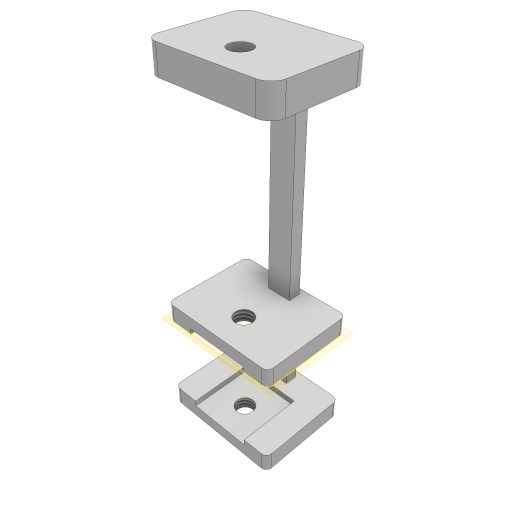
# Autodesk Inventor part: Crystal-Cut10x10-screwM4
Saved by Autodesk Inventor 2023 (Build 270158000, 158)
## iProperties
Created: 2021-08-04
Part Number: Crystal-Cut10x10-screwM4
Material: Generic
Document SubType Name: Modeling
Designer: Nikita
Density: 1 g/cm^3
Appearance: Default
Author: Nikita
Autodesk Inventor part; units mm, degrees
ref_plane "YZ Plane" through (0, 0, 0) normal (1, 0, 0) x (0, 1, 0)
ref_plane "XZ Plane" through (0, 0, 0) normal (0, 1, 0) x (-1, 0, 0)
ref_plane "XY Plane" through (0, 0, 0) normal (0, 0, 1) x (1, 0, 0)
sketch "Sketch1" plane through (0, 0, 0) normal (0, 0, 1) x (1, 0, 0)
  line L0 (0, 0) -> (19, 0)
  line L1 (19, 0) -> (19, 15)
  line L2 (19, 15) -> (0, 15)
  line L3 (0, 15) -> (0, 0)
  point P0 (9.5, 15)
  dimension "d0" = 19
  dimension "d1" = 15
  constraints: 8 end point, 2 parallel, 1 horizontal, 1 midpoint, 1 perpendicular
  measures "d0" distance of L2.end L1.end
  measures "d1" distance of L1.end L0.end
extrude "Extrusion1" add sketch "Sketch1" along normal blind 3
sketch "Sketch2" plane through (0, 0, 3) normal (0, 0, 1) x (1, 0, 0)
  line L0 (19, 15) -> (0, 15) projected
  circle A0 centre (9.5, 13) radius 1
  point P0 (0, 0)
  point P1 (9.5, 15)
  dimension "d4" = 2
  dimension "d5" = 2
  constraints: 1 centre point, 1 midpoint
  measures "d4" diameter of A0
  measures "d5" distance from line of A0.centre L0
extrude "Extrusion2" add sketch "Sketch2" along normal blind 1.5
sketch "Sketch6" plane through (9.5, 13, 4.5) normal (0, 0, 1) x (1, 0, 0)
  circle A0 centre (0, 0) radius 1 projected
  line L0 (2, -1) -> (-2, -1)
  line L1 (-2, -1) -> (-2, 1)
  line L2 (-2, 1) -> (2, 1)
  line L3 (2, 1) -> (2, -1)
  line L4 (2, -1) -> (-2, 1) construction
  line L5 (-2, -1) -> (2, 1) construction
  point P0 (-9.5, -13)
  dimension "d13" = 4
  constraints: 12 end point, 2 midpoint, 2 parallel, 1 coincident, 1 horizontal, 1 perpendicular
  measures "d13" distance of L1.end L2.end
extrude "Extrusion5" add sketch "Sketch6" along normal blind 47
sketch "Sketch7" plane through (9.5, 13, 51.5) normal (0, 0, 1) x (1, 0, 0)
  circle A0 centre (0, 0) radius 1 projected
  line L0 (-9.5, -13) -> (9.5, -13) projected
  line L1 (9.5, -13) -> (9.5, 2) projected
  line L2 (9.5, 2) -> (-9.5, 2) projected
  line L3 (-9.5, 2) -> (-9.5, -13) projected
  arc A1 (0, -1) -> (0, 1) centre (0, 0) ccw projected
  arc A2 (0, 1) -> (0, -1) centre (0, 0) ccw projected
extrude "Extrusion6" add sketch "Sketch7" along normal blind 4 contours A0 | L3 L2 L1 L0
fillet "Fillet2" radius 1 4 edges at (19, 0, 1.5) (19, 15, 1.5) (0, 0, 1.5) (0, 15, 1.5)
fillet "Fillet3" radius 2 4 edges at (19, 0, 53.5) (19, 15, 53.5) (0, 0, 53.5) (0, 15, 53.5)
extrude "Extrusion10" add sketch "Sketch6" against normal up to surface (1.5 mm away) contours A0 L2 L3 L0 | A0 L0 L1 L2
sketch "Sketch13" plane through (0, 0, 3) normal (0, 0, 1) x (1, 0, 0)
  line L0 (11.5, 12) -> (7.5, 12) projected
  line L1 (7.5, 12) -> (7.5, 14) projected
  line L2 (7.5, 14) -> (11.5, 14) projected
  line L3 (11.5, 14) -> (11.5, 12) projected
  arc A0 (1, 15) -> (0, 14) centre (1, 14) ccw projected
  line L4 (0, 14) -> (0, 1) projected
  arc A1 (0, 1) -> (1, 0) centre (1, 1) ccw projected
  line L5 (1, 0) -> (18, 0) projected
  arc A2 (18, 0) -> (19, 1) centre (18, 1) ccw projected
  line L6 (19, 1) -> (19, 14) projected
  arc A3 (19, 14) -> (18, 15) centre (18, 14) ccw projected
  line L7 (18, 15) -> (1, 15) projected
  line L8 (4.5, 10.2) -> (14.7, 10.2)
  line L9 (14.7, 10.2) -> (14.7, 0)
  line L10 (14.7, 0) -> (4.5, 0)
  line L11 (4.5, 0) -> (4.5, 10.2)
  point P0 (0, 0)
  point P1 (14.7, 0)
  dimension "d67" = 10.2
  dimension "d68" = 10.2
  dimension "d69" = 4.5
  constraints: 8 end point, 2 parallel, 1 collinear, 1 horizontal, 1 perpendicular
  measures "d67" distance of L9.end L10.end
  measures "d68" distance of L8.end L9.end
  measures "d69" distance between parallel lines of L4 L11
extrude "Extrusion12" cut sketch "Sketch13" against normal blind 1 contours L11 L8 L9 L5
ref_plane "Work Plane1" through (0, 0, 16) normal (0, 0, 1) x (1, 0, 0)
sketch "Sketch14" plane through (0, 0, 16) normal (0, 0, 1) x (1, 0, 0)
  line L0 (4.5, 0) -> (4.5, 10.2) projected
  line L1 (4.5, 10.2) -> (14.7, 10.2) projected
  line L2 (14.7, 10.2) -> (14.7, 0) projected
  line L3 (14.7, 0) -> (18, 0) projected
  arc A0 (18, 0) -> (19, 1) centre (18, 1) ccw projected
  line L4 (19, 1) -> (19, 14) projected
  arc A1 (19, 14) -> (18, 15) centre (18, 14) ccw projected
  line L5 (18, 15) -> (1, 15) projected
  arc A2 (1, 15) -> (0, 14) centre (1, 14) ccw projected
  line L6 (0, 14) -> (0, 1) projected
  arc A3 (0, 1) -> (1, 0) centre (1, 1) ccw projected
  line L7 (1, 0) -> (4.5, 0) projected
  line L8 (11.5, 12) -> (7.5, 12) projected
  line L9 (7.5, 12) -> (7.5, 14) projected
  line L10 (7.5, 14) -> (11.5, 14) projected
  line L11 (11.5, 14) -> (11.5, 12) projected
  line L12 (4.5, 0) -> (4.5, 10.2) projected
  line L13 (14.7, 0) -> (4.5, 0) projected
  line L14 (14.7, 10.2) -> (14.7, 0) projected
  line L15 (4.5, 10.2) -> (14.7, 10.2) projected
  point P0 (0, 0)
extrude "Extrusion13" add sketch "Sketch14" along normal blind 3
sketch "Sketch15" plane through (0, 0, 19) normal (0, 0, 1) x (1, 0, 0)
  line L0 (4.5, 0) -> (4.5, 10.2) projected
  line L1 (14.7, 0) -> (4.5, 0) projected
  line L2 (14.7, 10.2) -> (14.7, 0) projected
  line L3 (4.5, 10.2) -> (14.7, 10.2) projected
  point P0 (0, 0)
  point P1 (9.6, 5.1)
hole "Hole1" at (9.6, 5.1, 19) direction (0, 0, -1) diameter 3.242 end through all thread size "M4x0.7" class "6H" standard "ISO Metric profile"
extrude "Extrusion14" cut sketch "Sketch14" along normal blind 1 contours L0 L1 L2 L13
sketch "Sketch16" plane through (9.5, 13, 55.5) normal (0, 0, 1) x (1, 0, 0)
  circle A0 centre (0.1, -7.9) radius 1.621 projected
  point P0 (-9.5, -13)
extrude "Extrusion15" cut sketch "Sketch16" against normal up to surface (4 mm away)
body "Solid1"
